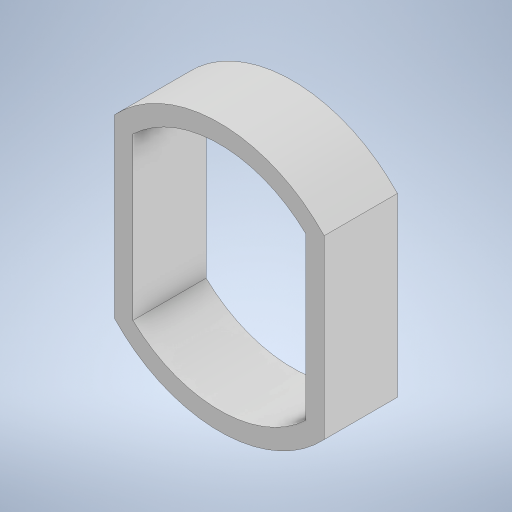
# Autodesk Inventor part: motor_holder_test_fit
Saved by Autodesk Inventor 2024 (Build 280153000, 153)
## iProperties
Created: 2024-05-25
Part Number: motor_holder_test_fit
Material: Generic
Document SubType Name: Modeling
Designer: david
Density: 1 g/cm^3
Appearance: Default
Author: david
Autodesk Inventor part; units mm, degrees
ref_plane "YZ Plane" through (0, 0, 0) normal (1, 0, 0) x (0, 1, 0)
ref_plane "XZ Plane" through (0, 0, 0) normal (0, 1, 0) x (-1, 0, 0)
ref_plane "XY Plane" through (0, 0, 0) normal (0, 0, 1) x (1, 0, 0)
sketch "Sketch1" plane through (0, 0, 0) normal (0, 0, 1) x (1, 0, 0)
  line L0 (0, 0) -> (15, 0)
  line L1 (15, 0) -> (15, 20)
  line L2 (15, 20) -> (0, 20)
  line L3 (0, 20) -> (0, 0)
  line L4 (0, 3) -> (15, 3)
  line L5 (15, 3) -> (15, 17)
  line L6 (15, 17) -> (0, 17)
  line L7 (0, 17) -> (0, 3)
  line L8 (0, 3) -> (15, 17) construction
  line L9 (15, 3) -> (0, 17) construction
  arc A0 (15, 17) -> (0, 17) centre (7.5, 9.125) ccw
  arc A1 (0, 3) -> (15, 3) centre (7.5, 10.875) ccw
  line L10 (-1.5875, -1.5875) -> (16.5875, -1.5875)
  line L11 (16.5875, -1.5875) -> (16.5875, 21.5875)
  line L12 (16.5875, 21.5875) -> (-1.5875, 21.5875)
  line L13 (-1.5875, 21.5875) -> (-1.5875, -1.5875)
  arc A2 (18.2337, 15.4576) -> (-3.6211, 14.7494) centre (7.5, 9.125) ccw
  line L14 (7.5, 10) -> (5.1883, 10)
  arc A3 (-3.6211, 5.2506) -> (18.2337, 4.5424) centre (7.5, 10.875) ccw
  point P0 (16.5875, 2.3467)
  point P1 (16.5875, 17.6533)
  point P2 (-1.5875, 17.6533)
  point P3 (-1.5875, 2.3467)
  dimension "d2" = 15
  dimension "d3" = 20
  dimension "d4" = 14
  dimension "d5" = 7.5
  dimension "d6" = 10
  dimension "d7" = 1.5875
  dimension "d8" = 1.5875
  constraints: 30 end point, 8 point on circle, 6 parallel, 4 centre point, 3 horizontal, 3 perpendicular, 3 symmetric about line, 2 coincident, 2 midpoint, 2 tangent, 1 point on line, 4 other
  measures "d2" distance of L2.end L1.end
  measures "d3" distance of L0.end L1.end
  measures "d4" distance of L5.end L4.end
  measures "d5" distance from line of L1 L14.start
  measures "d6" distance from line of L0 L14.start
  measures "d7" distance between parallel lines of L13 L7
  measures "d8" radial gap between concentric circles of A0 A2
extrude "Extrusion1" add sketch "Sketch1" along normal blind 6.35 contours A3 L3 A1 L0 | L0 A3 | A3 L13 A2 L3 | A1 L1 A3 L0 | L1 A2 L11 A3 | L3 A2 L2 A0 | A0 L2 A2 L1 | L2 A2
body "Solid1"
